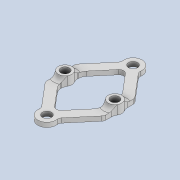
# Autodesk Inventor part: enc_t_hh
Saved by Autodesk Inventor 2020 (Build 240168000, 168)
## iProperties
Created: 2021-09-18
Part Number: enc_t_hh
Material: Generic
Document SubType Name: Modeling
Designer: Shuang Peng
Density: 1 g/cm^3
Appearance: Default
Author: Shuang Peng
Autodesk Inventor part; units mm, degrees
ref_plane "YZ Plane" through (0, 0, 0) normal (1, 0, 0) x (0, 1, 0)
ref_plane "XZ Plane" through (0, 0, 0) normal (0, 1, 0) x (-1, 0, 0)
ref_plane "XY Plane" through (0, 0, 0) normal (0, 0, 1) x (1, 0, 0)
sketch "Sketch1" plane through (0, 0, 0) normal (0, 1, 0) x (-1, 0, 0)
  line L0 (0, 0) -> (0, -19)
  line L1 (0, -9.5) -> (5.5, -9.5)
  line L2 (0, -9.5) -> (-5.5, -9.5)
  line L3 (5.5, -6.5) -> (5.5, -12.5) construction
  line L4 (4.5, -6.5) -> (4.5, -12.5)
  line L5 (6.5, -12.5) -> (6.5, -6.5)
  arc A0 (6.5, -6.5) -> (4.5, -6.5) centre (5.5, -6.5) ccw
  arc A1 (4.5, -12.5) -> (6.5, -12.5) centre (5.5, -12.5) ccw
  line L6 (-5.5, -6.5) -> (-5.5, -12.5) construction
  line L7 (-6.5, -6.5) -> (-6.5, -12.5)
  line L8 (-4.5, -12.5) -> (-4.5, -6.5)
  arc A2 (-4.5, -6.5) -> (-6.5, -6.5) centre (-5.5, -6.5) ccw
  arc A3 (-6.5, -12.5) -> (-4.5, -12.5) centre (-5.5, -12.5) ccw
  line L9 (0, 0) -> (5.5, -6.5) construction
  line L10 (-0.763386, -0.645942) -> (4.736614, -7.145942)
  line L11 (6.263386, -5.854058) -> (0.763386, 0.645942)
  arc A4 (0.763386, 0.645942) -> (-0.763386, -0.645942) centre (0, 0) ccw
  arc A5 (4.736614, -7.145942) -> (6.263386, -5.854058) centre (5.5, -6.5) ccw
  line L12 (5.5, -12.5) -> (0, -19) construction
  line L13 (4.736614, -11.854058) -> (-0.763386, -18.354058)
  line L14 (0.763386, -19.645942) -> (6.263386, -13.145942)
  arc A6 (6.263386, -13.145942) -> (4.736614, -11.854058) centre (5.5, -12.5) ccw
  arc A7 (-0.763386, -18.354058) -> (0.763386, -19.645942) centre (0, -19) ccw
  line L15 (-5.5, -6.5) -> (0, 0) construction
  line L16 (-4.736614, -7.145942) -> (0.763386, -0.645942)
  line L17 (-0.763386, 0.645942) -> (-6.263386, -5.854058)
  arc A8 (-6.263386, -5.854058) -> (-4.736614, -7.145942) centre (-5.5, -6.5) ccw
  arc A9 (0.763386, -0.645942) -> (-0.763386, 0.645942) centre (0, 0) ccw
  line L18 (-5.5, -12.5) -> (0, -19) construction
  line L19 (-4.736614, -11.854058) -> (0.763386, -18.354058)
  line L20 (-0.763386, -19.645942) -> (-6.263386, -13.145942)
  arc A10 (-4.736614, -11.854058) -> (-6.263386, -13.145942) centre (-5.5, -12.5) ccw
  arc A11 (-0.763386, -19.645942) -> (0.763386, -18.354058) centre (0, -19) ccw
  circle A12 centre (0, 0) radius 2
  circle A13 centre (5.5, -9.5) radius 1.5
  circle A14 centre (-5.5, -9.5) radius 1.5
  circle A15 centre (0, -19) radius 2
  point P0 (2.75, -3.25)
  point P1 (2.75, -15.75)
  point P2 (-2.75, -3.25)
  point P3 (-2.75, -15.75)
  point P4 (-4.5, -6.866308)
  point P5 (-0.355418, -1.968166)
  point P6 (0.355418, -1.968166)
  point P7 (4.5, -6.866308)
  point P8 (4.5, -8.381966)
  point P9 (4.5, -10.618034)
  point P10 (4.5, -12.133692)
  point P11 (0.355418, -17.031834)
  point P12 (-0.355418, -17.031834)
  point P13 (-4.5, -12.133692)
  point P14 (-4.5, -10.618034)
  point P15 (-4.5, -8.381966)
  point P16 (-6.5, -8.381966)
  point P17 (-6.5, -10.618034)
  point P18 (-1.882191, -18.323718)
  point P19 (1.882191, -18.323718)
  point P20 (6.5, -10.618034)
  point P21 (6.5, -8.381966)
  point P22 (1.882191, -0.676282)
  point P23 (-1.882191, -0.676282)
  dimension "d0" = 19
  dimension "d1" = 5.5
  dimension "d2" = 5.5
  dimension "d3" = 3
  dimension "d4" = 2
  dimension "d5" = 3
  dimension "d6" = 2
  dimension "d7" = 2
  dimension "d8" = 2
  dimension "d9" = 1
  dimension "d10" = 1
  dimension "d11" = 4
  dimension "d12" = 3
  dimension "d13" = 3
  dimension "d14" = 4
  constraints: 54 end point, 24 point on circle, 24 tangent, 16 centre point, 7 midpoint, 6 parallel, 4 coincident, 2 horizontal, 2 vertical, 1 concentric, 1 perpendicular
  measures "d0" distance of L0.start L0.end
  measures "d1" distance of L1.start L1.end
  measures "d2" distance of L1.start L2.end
  measures "d3" distance of L1.end L3.end
  measures "d4" diameter of A1
  measures "d5" distance of L2.end L6.end
  measures "d6" diameter of A3
  measures "d7" diameter of A5
  measures "d8" diameter of A7
  measures "d9" radius of A10
  measures "d10" radius of A8
  measures "d11" diameter of A12
  measures "d12" diameter of A13
  measures "d13" diameter of A14
  measures "d14" diameter of A15
extrude "Extrusion1" add sketch "Sketch1" along normal blind 1 contours L10 A12 L0 | L16 A12 L17 A4 L10 | L16 A9 L11 A12 L10 | L0 A12 L16 | L10 A4 A9 L16 | A12 L11 A0 L4 L10 | L16 L8 A2 L17 A12 | L17 A12 L11 A4 | L10 A5 L5 A13 L4 | L4 A0 A5 L10 | L16 A8 A2 L8 | L8 A14 L7 A8 L16 | A15 L13 L0 | L0 L19 A15 | A13 L4 L1 | L1 L4 A13 | A14 L8 L2 | L2 L8 A14 | A13 L5 L4 | L8 A14 L7 | L19 A11 A7 L13 | L13 A7 L20 A15 L19 | L13 A15 L14 A11 L19 | L13 L4 A1 L14 A15 | A15 L20 A3 L8 L19 | A13 L5 A6 L13 L4 | L8 L19 A10 L7 A14 | A13 L5 | L7 A14 | L13 A6 A1 L4 | A15 L20 A7 L14 | L8 A3 A10 L19
sketch "Sketch2" plane through (0, 1, 0) normal (0, 1, 0) x (1, 0, 0)
  arc A0 (-1.882191, 0.676282) -> (1.882191, 0.676282) centre (0, 0) ccw
  line L0 (1.882191, 0.676282) -> (6.263386, 5.854058)
  arc A1 (6.263386, 5.854058) -> (6.5, 6.5) centre (5.5, 6.5) ccw
  line L1 (6.5, 6.5) -> (6.5, 8.381966)
  arc A2 (6.5, 8.381966) -> (6.5, 10.618034) centre (5.5, 9.5) ccw
  line L2 (6.5, 10.618034) -> (6.5, 12.5)
  arc A3 (6.5, 12.5) -> (6.263386, 13.145942) centre (5.5, 12.5) ccw
  line L3 (6.263386, 13.145942) -> (1.882191, 18.323718)
  arc A4 (1.882191, 18.323718) -> (-1.882191, 18.323718) centre (0, 19) ccw
  line L4 (-1.882191, 18.323718) -> (-6.263386, 13.145942)
  arc A5 (-6.263386, 13.145942) -> (-6.5, 12.5) centre (-5.5, 12.5) ccw
  line L5 (-6.5, 12.5) -> (-6.5, 10.618034)
  arc A6 (-6.5, 10.618034) -> (-6.5, 8.381966) centre (-5.5, 9.5) ccw
  line L6 (-6.5, 8.381966) -> (-6.5, 6.5)
  arc A7 (-6.5, 6.5) -> (-6.263386, 5.854058) centre (-5.5, 6.5) ccw
  line L7 (-6.263386, 5.854058) -> (-1.882191, 0.676282)
  line L8 (-0.355418, 1.968166) -> (-4.5, 6.866308)
  line L9 (-4.5, 6.866308) -> (-4.5, 8.381966)
  arc A8 (-4.5, 8.381966) -> (-4.5, 10.618034) centre (-5.5, 9.5) ccw
  line L10 (-4.5, 10.618034) -> (-4.5, 12.133692)
  line L11 (-4.5, 12.133692) -> (-0.355418, 17.031834)
  arc A9 (-0.355418, 17.031834) -> (0.355418, 17.031834) centre (0, 19) ccw
  line L12 (0.355418, 17.031834) -> (4.5, 12.133692)
  line L13 (4.5, 12.133692) -> (4.5, 10.618034)
  arc A10 (4.5, 10.618034) -> (4.5, 8.381966) centre (5.5, 9.5) ccw
  line L14 (4.5, 8.381966) -> (4.5, 6.866308)
  line L15 (4.5, 6.866308) -> (0.355418, 1.968166)
  arc A11 (0.355418, 1.968166) -> (-0.355418, 1.968166) centre (0, 0) ccw
hole "Hole1" at (-5.5, 1, -9.5) at (5.5, 1, -9.5) direction (0, -1, 0) diameter 1.9 depth 100
sketch "Sketch3" plane through (0, 1, 0) normal (0, 1, 0) x (1, 0, 0)
  circle A0 centre (-5.5, 9.5) radius 0.95
  circle A1 centre (5.5, 9.5) radius 0.95
  arc A2 (-1.882191, 0.676282) -> (1.882191, 0.676282) centre (0, 0) ccw
  line L0 (1.882191, 0.676282) -> (6.263386, 5.854058)
  arc A3 (6.263386, 5.854058) -> (6.5, 6.5) centre (5.5, 6.5) ccw
  line L1 (6.5, 6.5) -> (6.5, 8.381966)
  arc A4 (6.5, 8.381966) -> (6.5, 10.618034) centre (5.5, 9.5) ccw
  line L2 (6.5, 10.618034) -> (6.5, 12.5)
  arc A5 (6.5, 12.5) -> (6.263386, 13.145942) centre (5.5, 12.5) ccw
  line L3 (6.263386, 13.145942) -> (1.882191, 18.323718)
  arc A6 (1.882191, 18.323718) -> (-1.882191, 18.323718) centre (0, 19) ccw
  line L4 (-1.882191, 18.323718) -> (-6.263386, 13.145942)
  arc A7 (-6.263386, 13.145942) -> (-6.5, 12.5) centre (-5.5, 12.5) ccw
  line L5 (-6.5, 12.5) -> (-6.5, 10.618034)
  arc A8 (-6.5, 10.618034) -> (-6.5, 8.381966) centre (-5.5, 9.5) ccw
  line L6 (-6.5, 8.381966) -> (-6.5, 6.5)
  arc A9 (-6.5, 6.5) -> (-6.263386, 5.854058) centre (-5.5, 6.5) ccw
  line L7 (-6.263386, 5.854058) -> (-1.882191, 0.676282)
  line L8 (-0.355418, 1.968166) -> (-4.5, 6.866308)
  line L9 (-4.5, 6.866308) -> (-4.5, 8.381966)
  arc A10 (-4.5, 8.381966) -> (-4.5, 10.618034) centre (-5.5, 9.5) ccw
  line L10 (-4.5, 10.618034) -> (-4.5, 12.133692)
  line L11 (-4.5, 12.133692) -> (-0.355418, 17.031834)
  arc A11 (-0.355418, 17.031834) -> (0.355418, 17.031834) centre (0, 19) ccw
  line L12 (0.355418, 17.031834) -> (4.5, 12.133692)
  line L13 (4.5, 12.133692) -> (4.5, 10.618034)
  arc A12 (4.5, 10.618034) -> (4.5, 8.381966) centre (5.5, 9.5) ccw
  line L14 (4.5, 8.381966) -> (4.5, 6.866308)
  line L15 (4.5, 6.866308) -> (0.355418, 1.968166)
  arc A13 (0.355418, 1.968166) -> (-0.355418, 1.968166) centre (0, 0) ccw
hole "Hole2" at (0, 1, -19) at (0, 1, 0) direction (0, -1, 0) diameter 2 depth 100
sketch "Sketch4" plane through (0, 1, 0) normal (0, 1, 0) x (1, 0, 0)
  circle A0 centre (0, 19) radius 1
  circle A1 centre (0, 0) radius 1
  circle A2 centre (-5.5, 9.5) radius 0.95
  circle A3 centre (5.5, 9.5) radius 0.95
  arc A4 (-1.882191, 0.676282) -> (1.882191, 0.676282) centre (0, 0) ccw
  line L0 (1.882191, 0.676282) -> (6.263386, 5.854058)
  arc A5 (6.263386, 5.854058) -> (6.5, 6.5) centre (5.5, 6.5) ccw
  line L1 (6.5, 6.5) -> (6.5, 8.381966)
  arc A6 (6.5, 8.381966) -> (6.5, 10.618034) centre (5.5, 9.5) ccw
  line L2 (6.5, 10.618034) -> (6.5, 12.5)
  arc A7 (6.5, 12.5) -> (6.263386, 13.145942) centre (5.5, 12.5) ccw
  line L3 (6.263386, 13.145942) -> (1.882191, 18.323718)
  arc A8 (1.882191, 18.323718) -> (-1.882191, 18.323718) centre (0, 19) ccw
  line L4 (-1.882191, 18.323718) -> (-6.263386, 13.145942)
  arc A9 (-6.263386, 13.145942) -> (-6.5, 12.5) centre (-5.5, 12.5) ccw
  line L5 (-6.5, 12.5) -> (-6.5, 10.618034)
  arc A10 (-6.5, 10.618034) -> (-6.5, 8.381966) centre (-5.5, 9.5) ccw
  line L6 (-6.5, 8.381966) -> (-6.5, 6.5)
  arc A11 (-6.5, 6.5) -> (-6.263386, 5.854058) centre (-5.5, 6.5) ccw
  line L7 (-6.263386, 5.854058) -> (-1.882191, 0.676282)
  line L8 (-0.355418, 1.968166) -> (-4.5, 6.866308)
  line L9 (-4.5, 6.866308) -> (-4.5, 8.381966)
  arc A12 (-4.5, 8.381966) -> (-4.5, 10.618034) centre (-5.5, 9.5) ccw
  line L10 (-4.5, 10.618034) -> (-4.5, 12.133692)
  line L11 (-4.5, 12.133692) -> (-0.355418, 17.031834)
  arc A13 (-0.355418, 17.031834) -> (0.355418, 17.031834) centre (0, 19) ccw
  line L12 (0.355418, 17.031834) -> (4.5, 12.133692)
  line L13 (4.5, 12.133692) -> (4.5, 10.618034)
  arc A14 (4.5, 10.618034) -> (4.5, 8.381966) centre (5.5, 9.5) ccw
  line L14 (4.5, 8.381966) -> (4.5, 6.866308)
  line L15 (4.5, 6.866308) -> (0.355418, 1.968166)
  arc A15 (0.355418, 1.968166) -> (-0.355418, 1.968166) centre (0, 0) ccw
  circle A16 centre (-5.5, 9.5) radius 1.5
  circle A17 centre (5.5, 9.5) radius 0.95
  circle A18 centre (5.5, 9.5) radius 1.5
  point P0 (-6.5, 8.381966)
  dimension "d31" = 3
  dimension "d32" = 3
  constraints: 2 centre point, 2 coincident
  measures "d31" diameter of A16
  measures "d32" diameter of A18
extrude "Extrusion2" add sketch "Sketch4" along normal blind 1 contours A10 A16 A12 | A18 A14 A6
fillet "Fillet1" radius 2 12 edges at (4.5, 0.5, -8.382) (4.5, 0.5, -10.618) (4.5, 0.5, -12.1337) (4.5, 0.5, -6.8663) (6.5, 0.5, -8.382) (6.5, 0.5, -10.618) (-4.5, 0.5, -6.8663) (-4.5, 0.5, -8.382) (-4.5, 0.5, -10.618) (-4.5, 0.5, -12.1337) (-6.5, 0.5, -8.382) (-6.5, 0.5, -10.618)
fillet "Fillet2" radius 1 8 edges at (-6.6558, 1, -10.4561) (-5.5, 1, -11) (-4.3442, 1, -10.4561) (-5.5, 1, -8) (4.3442, 1, -10.4561) (5.5, 1, -11) (6.6558, 1, -10.4561) (5.5, 1, -8)
fillet "Fillet3" radius 1 8 edges at (-1.8822, 0.5, -0.6763) (1.8822, 0.5, -0.6763) (-0.3554, 0.5, -1.9682) (0.3554, 0.5, -1.9682) (-1.8822, 0.5, -18.3237) (1.8822, 0.5, -18.3237) (-0.3554, 0.5, -17.0318) (0.3554, 0.5, -17.0318)
body "Solid1"
